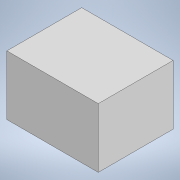
# Autodesk Inventor part: conector_ceramico
Saved by Autodesk Inventor 2021 (Build 250183000, 183)
## iProperties
Created: 2021-04-17
Part Number: conector_ceramico
Material: Genérico
Document SubType Name: Modeling
Designer: Leonardo Fabio Mercado Benítez
Density: 1 g/cm^3
Appearance: Valor por defecto
Author: Leonardo Fabio Mercado Benítez
Autodesk Inventor part; units mm, degrees
ref_plane "YZ Plane" through (0, 0, 0) normal (1, 0, 0) x (0, 1, 0)
ref_plane "XZ Plane" through (0, 0, 0) normal (0, 1, 0) x (-1, 0, 0)
ref_plane "XY Plane" through (0, 0, 0) normal (0, 0, 1) x (1, 0, 0)
sketch "Boceto1" plane through (0, 0, 0) normal (0, 1, 0) x (-1, 0, 0)
  line L0 (10.75, 8.8) -> (-10.75, 8.8)
  line L1 (-10.75, 8.8) -> (-10.75, -8.8)
  line L2 (-10.75, -8.8) -> (10.75, -8.8)
  line L3 (10.75, -8.8) -> (10.75, 8.8)
  line L4 (10.75, 8.8) -> (-10.75, -8.8) construction
  line L5 (-10.75, 8.8) -> (10.75, -8.8) construction
  point P0 (0, 0)
  dimension "d0" = 21.5
  dimension "d1" = 17.6
  constraints: 12 end point, 2 midpoint, 2 parallel, 1 horizontal, 1 perpendicular
  measures "d0" distance of L2.end L1.end
  measures "d1" distance of L1.end L0.end
extrude "Extrusión1" add sketch "Boceto1" along normal blind 14
